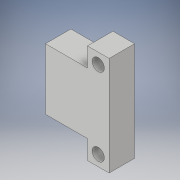
# Autodesk Inventor part: OPB732
Saved by Autodesk Inventor 2018 (Build 220112000, 112)
## iProperties
Created: 2018-03-26
Part Number: OPB732
Material: Generisch
Document SubType Name: Modeling
Designer: Julian
Density: 1 g/cm^3
Appearance: Vorgabe
Author: Julian
Autodesk Inventor part; units mm, degrees
ref_plane "YZ Plane" through (0, 0, 0) normal (1, 0, 0) x (0, 1, 0)
ref_plane "XZ Plane" through (0, 0, 0) normal (0, 1, 0) x (-1, 0, 0)
ref_plane "XY Plane" through (0, 0, 0) normal (0, 0, 1) x (1, 0, 0)
sketch "Skizze1" plane through (0, 0, 0) normal (0, 1, 0) x (-1, 0, 0)
  line L0 (0, 0) -> (4.32, 0)
  line L1 (4.32, 0) -> (4.32, -3.81)
  line L2 (4.32, -3.81) -> (12.7, -3.81)
  line L3 (12.7, -3.81) -> (12.7, -16)
  line L4 (12.7, -16) -> (4.32, -16)
  line L5 (4.32, -16) -> (4.32, -19.81)
  line L6 (4.32, -19.81) -> (0, -19.81)
  line L7 (0, -19.81) -> (0, 0)
  line L8 (2.16, 0) -> (2.16, -2.16)
  line L9 (2.16, -19.81) -> (2.16, -17.65)
  circle A0 centre (2.16, -2.16) radius 1.22
  circle A1 centre (2.16, -17.65) radius 1.22
  dimension "d0" = 4.32
  dimension "d1" = 3.81
  dimension "d2" = 8.38
  dimension "d3" = 12.19
  dimension "d4" = 3.81
  dimension "d5" = 2.16
  dimension "d6" = 2.16
  dimension "d7" = 2.44
  dimension "d8" = 2.44
  constraints: 20 end point, 6 perpendicular, 2 centre point, 2 coincident, 2 midpoint, 2 point on line, 2 vertical, 1 horizontal
  measures "d0" distance of L0.start L0.end
  measures "d1" distance of L0.end L1.end
  measures "d2" distance of L1.end L2.end
  measures "d3" distance of L2.end L3.end
  measures "d4" distance of L4.end L5.end
  measures "d5" distance of L8.start L8.end
  measures "d6" distance of L9.start L9.end
  measures "d7" diameter of A0
  measures "d8" diameter of A1
extrude "Extrusion1" add sketch "Skizze1" along normal blind 5.08
